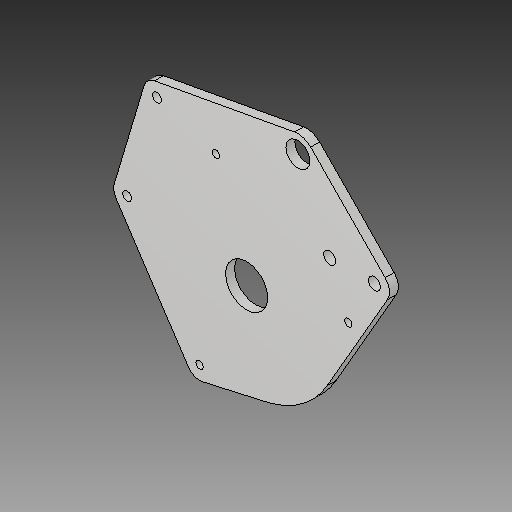
# Autodesk Inventor part: 前足内フレーム
Saved by Autodesk Inventor 2019 (Build 230136000, 136)
## iProperties
Created: 2019-09-17
Part Number: 前足内フレーム
Material: アルミニウム 2014-T4
Document SubType Name: Modeling
Designer: tanjihayato
Density: 2.8 g/cm^3
Appearance: サテン
Mass: 44.8961 g
Surface Area: 119.322 cm^2
Volume: 16.0343 cm^3
Author: tanjihayato
Autodesk Inventor part; units mm, degrees
ref_plane "YZ Plane" through (0, 0, 0) normal (1, 0, 0) x (0, 1, 0)
ref_plane "XZ Plane" through (0, 0, 0) normal (0, 1, 0) x (-1, 0, 0)
ref_plane "XY Plane" through (0, 0, 0) normal (0, 0, 1) x (1, 0, 0)
sketch "スケッチ3" plane through (0, 0, 0) normal (0, 0, 1) x (1, 0, 0)
  circle A0 centre (110.4743, -16.4118) radius 30.1 construction
  circle A1 centre (150.4743, 0.5882) radius 1.5
  circle A2 centre (127.6431, 30.2622) radius 1.5
  circle A3 centre (80.4743, 23.124) radius 1.5
  circle A4 centre (70.4743, -10.4118) radius 1.5
  circle A5 centre (110.4743, -16.4118) radius 7.025
  arc A6 (79.801, 27.5733) -> (76.162, 24.4099) centre (80.4743, 23.124) ccw
  arc A7 (131.2097, 33.0062) -> (126.9698, 34.7115) centre (127.6431, 30.2622) ccw
  arc A8 (154.401, -1.6098) -> (154.0408, 3.3323) centre (150.4743, 0.5882) ccw
  arc A9 (66.162, -9.1259) -> (66.7172, -12.8885) centre (70.4743, -10.4118) ccw
  arc A10 (117.3199, -46.749) -> (137.6119, -31.6026) centre (110.4743, -16.4118) ccw
  line L0 (154.401, -1.6098) -> (137.6119, -31.6026)
  line L1 (66.162, -9.1259) -> (76.162, 24.4099)
  line L2 (79.801, 27.5733) -> (126.9698, 34.7115)
  line L3 (131.2097, 33.0062) -> (154.0408, 3.3323)
  line L4 (96.5433, 16.3458) -> (118.2214, -10.0492) construction
  line L5 (117.0311, -23.9953) -> (91.1935, -46.3348) construction
  circle A11 centre (100.1953, 16.6261) radius 3 construction
  circle A12 centre (144.4932, -10.0968) radius 3 construction
  circle A13 centre (100.1953, 16.6261) radius 4.5 construction
  circle A14 centre (144.4932, -10.0968) radius 4.5 construction
  arc A15 (90.988, -49.7066) -> (95.7356, -51.6195) centre (94.7451, -47.2298) ccw
  circle A16 centre (94.7451, -47.2298) radius 3 construction
  line L6 (95.7356, -51.6195) -> (117.3199, -46.749)
  line L7 (66.7172, -12.8885) -> (90.988, -49.7066)
  circle A17 centre (100.1953, 16.6261) radius 1.25
  circle A18 centre (144.4932, -10.0968) radius 1.25
  circle A19 centre (94.7451, -47.2298) radius 1.25
  circle A20 centre (110.4743, -16.4118) radius 30.1 construction
  circle A21 centre (150.4743, 0.5882) radius 1.5
  circle A22 centre (127.6431, 30.2622) radius 1.5
  circle A23 centre (80.4743, 23.124) radius 1.5
  circle A24 centre (70.4743, -10.4118) radius 1.5
  circle A25 centre (110.4743, -16.4118) radius 7.025
  arc A26 (79.801, 27.5733) -> (76.162, 24.4099) centre (80.4743, 23.124) ccw
  arc A27 (131.2097, 33.0062) -> (126.9698, 34.7115) centre (127.6431, 30.2622) ccw
  arc A28 (154.401, -1.6098) -> (154.0408, 3.3323) centre (150.4743, 0.5882) ccw
  arc A29 (66.162, -9.1259) -> (66.7172, -12.8885) centre (70.4743, -10.4118) ccw
  arc A30 (117.3199, -46.749) -> (137.6119, -31.6026) centre (110.4743, -16.4118) ccw
  line L8 (154.401, -1.6098) -> (137.6119, -31.6026)
  line L9 (66.162, -9.1259) -> (76.162, 24.4099)
  line L10 (79.801, 27.5733) -> (126.9698, 34.7115)
  line L11 (131.2097, 33.0062) -> (154.0408, 3.3323)
  line L12 (96.5433, 16.3458) -> (118.2214, -10.0492) construction
  line L13 (117.0311, -23.9953) -> (91.1935, -46.3348) construction
  circle A31 centre (100.1953, 16.6261) radius 3 construction
  circle A32 centre (144.4932, -10.0968) radius 3 construction
  circle A33 centre (100.1953, 16.6261) radius 4.5 construction
  circle A34 centre (144.4932, -10.0968) radius 4.5 construction
  arc A35 (90.988, -49.7066) -> (95.7356, -51.6195) centre (94.7451, -47.2298) ccw
  circle A36 centre (94.7451, -47.2298) radius 3 construction
  line L14 (95.7356, -51.6195) -> (117.3199, -46.749)
  line L15 (66.7172, -12.8885) -> (90.988, -49.7066)
  circle A37 centre (100.1953, 16.6261) radius 1.25
  circle A38 centre (144.4932, -10.0968) radius 1.25
  circle A39 centre (94.7451, -47.2298) radius 1.25
  circle A40 centre (153.2732, 5.5882) radius 1.5
  circle A41 centre (138.2732, 5.5882) radius 1.5
  arc A42 (157.1998, 3.3902) -> (156.3941, 8.8301) centre (153.2732, 5.5882) ccw
  line L16 (154.401, -1.6098) -> (157.1998, 3.3902)
  line L17 (130.7641, 33.504) -> (156.3941, 8.8301)
  circle A43 centre (138.2732, 5.5882) radius 3
  circle A44 centre (153.2732, 5.5882) radius 3
  point P0 (0, 0)
  point P1 (0, 0)
  point P2 (0, 0)
  dimension "d20" = 14.05
  dimension "d21" = 9
  dimension "d22" = 9
  dimension "d23" = 9
  dimension "d24" = 9
  dimension "d25" = 1
  dimension "d26" = 6
  dimension "d27" = 6
  dimension "d28" = 9
  dimension "d29" = 9
  dimension "d30" = 9
  dimension "d31" = 6
  dimension "d32" = 2.5
  dimension "d33" = 2.5
  dimension "d34" = 2.5
  dimension "d37" = 14.05
  dimension "d38" = 9
  dimension "d39" = 9
  dimension "d40" = 9
  dimension "d41" = 9
  dimension "d42" = 1
  dimension "d43" = 6
  dimension "d44" = 6
  dimension "d45" = 9
  dimension "d46" = 9
  dimension "d47" = 9
  dimension "d48" = 6
  dimension "d49" = 2.5
  dimension "d50" = 2.5
  dimension "d51" = 2.5
  dimension "d52" = 3
  dimension "d53" = 3
  dimension "d54" = 15
  dimension "d55" = 9
  dimension "d56" = 6
  dimension "d57" = 6
  dimension "d58" = 5
  constraints: 45 centre point, 39 tangent, 36 end point, 27 coincident, 27 point on circle, 1 collinear, 1 horizontal alignment
  measures "d20" diameter of A5
  measures "d21" diameter of A6
  measures "d22" diameter of A7
  measures "d23" diameter of A8
  measures "d24" diameter of A9
  measures "d25" radial gap between concentric circles of A10 A0
  measures "d26" diameter of A11
  measures "d27" diameter of A12
  measures "d28" diameter of A13
  measures "d29" diameter of A14
  measures "d30" diameter of A15
  measures "d31" diameter of A16
  measures "d32" diameter of A17
  measures "d33" diameter of A18
  measures "d34" diameter of A19
  measures "d37" diameter of A25
  measures "d38" diameter of A26
  measures "d39" diameter of A27
  measures "d40" diameter of A28
  measures "d41" diameter of A29
  measures "d42" radial gap between concentric circles of A30 A20
  measures "d43" diameter of A31
  measures "d44" diameter of A32
  measures "d45" diameter of A33
  measures "d46" diameter of A34
  measures "d47" diameter of A35
  measures "d48" diameter of A36
  measures "d49" diameter of A37
  measures "d50" diameter of A38
  measures "d51" diameter of A39
  measures "d52" diameter of A40
  measures "d53" diameter of A41
  measures "d54" distance of A41.centre A40.centre
  measures "d55" diameter of A42
  measures "d56" diameter of A43
  measures "d57" diameter of A44
  measures "d58" vertical distance of A21.centre A40.centre
extrude "押し出し3" add sketch "スケッチ3" along normal blind 3 contours A1 | L2 A7 L3 A44 A8 L0 A10 L6 A15 L7 A9 L1 A6 | L17 A42 L16 A8 A44 L3 A7 | A44 A8 L3 A40 | L3 A40 A8 A44 | A40 L3 | L3 A40 | A43
extrude "押し出し4" cut sketch "スケッチ3" along normal blind 10 contours A40 L3 | L3 A40
sketch "スケッチ4" plane through (0, 0, 3) normal (0, 0, 1) x (1, 0, 0)
  circle A0 centre (153.2732, 5.5882) radius 1.5 projected
  circle A1 centre (138.2732, 5.5882) radius 1.5 projected
  circle A2 centre (110.4743, -16.4118) radius 7.025 projected
  circle A3 centre (70.4743, -10.4118) radius 1.5 projected
  circle A4 centre (80.4743, 23.124) radius 1.5 projected
  circle A5 centre (127.6431, 30.2622) radius 1.5 projected
  circle A6 centre (94.7451, -47.2298) radius 1.25 projected
  circle A7 centre (144.4932, -10.0968) radius 1.25 projected
  circle A8 centre (100.1953, 16.6261) radius 1.25 projected
  arc A9 (79.801, 27.5733) -> (76.162, 24.4099) centre (80.4743, 23.124) ccw projected
  line L0 (76.162, 24.4099) -> (66.162, -9.1259) projected
  arc A10 (66.162, -9.1259) -> (66.7172, -12.8885) centre (70.4743, -10.4118) ccw projected
  line L1 (66.7172, -12.8885) -> (90.988, -49.7066) projected
  arc A11 (90.988, -49.7066) -> (95.7356, -51.6195) centre (94.7451, -47.2298) ccw projected
  line L2 (95.7356, -51.6195) -> (117.3199, -46.749) projected
  arc A12 (117.3199, -46.749) -> (137.6119, -31.6026) centre (110.4743, -16.4118) ccw projected
  line L3 (137.6119, -31.6026) -> (157.1998, 3.3902) projected
  arc A13 (157.1998, 3.3902) -> (156.3941, 8.8301) centre (153.2732, 5.5882) ccw projected
  line L4 (156.3941, 8.8301) -> (130.7641, 33.504) projected
  arc A14 (130.7641, 33.504) -> (126.9698, 34.7115) centre (127.6431, 30.2622) ccw projected
  line L5 (126.9698, 34.7115) -> (79.801, 27.5733) projected
  circle A15 centre (127.6431, 30.2622) radius 4.025
  arc A16 (131.983, 34.4054) -> (126.5593, 36.1635) centre (127.6431, 30.2622) ccw
  line L6 (79.6614, 27.5499) -> (126.5593, 36.1635)
  line L7 (131.983, 34.4054) -> (156.528, 8.6956)
  point P0 (0, 0)
  dimension "d61" = 8.05
  dimension "d62" = 12
  constraints: 4 end point, 4 point on circle, 4 tangent, 2 centre point, 2 coincident
  measures "d61" diameter of A15
  measures "d62" diameter of A16
extrude "押し出し5" add sketch "スケッチ4" against normal blind 3 contours A9 L6 A16 L7 A13 L4 A14 L5
extrude "押し出し6" cut sketch "スケッチ4" against normal blind 3 contours A15
sketch "スケッチ5" plane through (0, 0, 3) normal (0, 0, 1) x (1, 0, 0)
  circle A0 centre (127.6431, 30.2622) radius 4.025 projected
  circle A1 centre (153.2732, 5.5882) radius 1.5 projected
  circle A2 centre (138.2732, 5.5882) radius 1.5 projected
  circle A3 centre (110.4743, -16.4118) radius 7.025 projected
  circle A4 centre (70.4743, -10.4118) radius 1.5 projected
  circle A5 centre (80.4743, 23.124) radius 1.5 projected
  circle A6 centre (94.7451, -47.2298) radius 1.25 projected
  circle A7 centre (144.4932, -10.0968) radius 1.25 projected
  circle A8 centre (100.1953, 16.6261) radius 1.25 projected
  arc A9 (79.6614, 27.5499) -> (76.162, 24.4099) centre (80.4743, 23.124) ccw projected
  line L0 (76.162, 24.4099) -> (66.162, -9.1259) projected
  arc A10 (66.162, -9.1259) -> (66.7172, -12.8885) centre (70.4743, -10.4118) ccw projected
  line L1 (66.7172, -12.8885) -> (90.988, -49.7066) projected
  arc A11 (90.988, -49.7066) -> (95.7356, -51.6195) centre (94.7451, -47.2298) ccw projected
  line L2 (95.7356, -51.6195) -> (117.3199, -46.749) projected
  arc A12 (117.3199, -46.749) -> (137.6119, -31.6026) centre (110.4743, -16.4118) ccw projected
  line L3 (137.6119, -31.6026) -> (157.1998, 3.3902) projected
  arc A13 (157.1998, 3.3902) -> (156.528, 8.6956) centre (153.2732, 5.5882) ccw projected
  line L4 (156.528, 8.6956) -> (131.983, 34.4054) projected
  arc A14 (131.983, 34.4054) -> (126.5593, 36.1635) centre (127.6431, 30.2622) ccw projected
  line L5 (126.5593, 36.1635) -> (79.6614, 27.5499) projected
  circle A15 centre (153.2732, 5.5882) radius 2
  circle A16 centre (138.2732, 5.5882) radius 2
  arc A17 (157.6055, 3.092) -> (156.8408, 9.0914) centre (153.2732, 5.5882) ccw
  line L6 (131.9243, 34.466) -> (156.8408, 9.0914)
  line L7 (157.6055, 3.092) -> (137.4212, -31.9384)
  arc A18 (117.3199, -46.749) -> (137.6119, -31.6026) centre (110.4743, -16.4118) ccw projected
  arc A19 (131.983, 34.4054) -> (126.5593, 36.1635) centre (127.6431, 30.2622) ccw projected
  point P0 (0, 0)
  dimension "d67" = 4
  dimension "d68" = 4
  dimension "d69" = 3
  constraints: 4 end point, 4 point on circle, 4 tangent, 3 centre point, 2 coincident
  measures "d67" diameter of A15
  measures "d68" diameter of A16
  measures "d69" radial gap between concentric circles of A15 A17
extrude "押し出し7" add sketch "スケッチ5" against normal blind 3 contours L6 A17 L7 A12 L3 A13 L4
extrude "押し出し8" cut sketch "スケッチ5" against normal blind 3 contours A15 | A16
